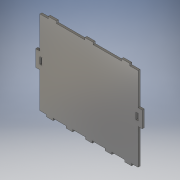
# Autodesk Inventor part: 1-8inch_Middle_2-Parts
Saved by Autodesk Inventor 2018 (Build 220112000, 112)
## iProperties
Created: 2018-01-26
Part Number: 1-8inch_Middle_2-Parts
Material: Generic
Document SubType Name: Modeling
Designer: Olivier
Density: 1 g/cm^3
Appearance: Default
Author: Olivier
Autodesk Inventor part; units mm, degrees
ref_plane "YZ Plane" through (0, 0, 0) normal (1, 0, 0) x (0, 1, 0)
ref_plane "XZ Plane" through (0, 0, 0) normal (0, 1, 0) x (-1, 0, 0)
ref_plane "XY Plane" through (0, 0, 0) normal (0, 0, 1) x (1, 0, 0)
sketch "Sketch1" plane through (0, 0, 0) normal (0, 0, 1) x (1, 0, 0)
  line L0 (-0.5, -5) -> (2.5, -5)
  line L1 (2.5, 5) -> (-0.5, 5)
  line L2 (-0.5, 5) -> (-0.5, -5)
  line L3 (-0.5, 12.5) -> (-0.5, 61.825)
  line L4 (19, 65) -> (24.9, 65)
  line L5 (69, 65) -> (79, 65)
  line L6 (124.9125, 65) -> (129, 65)
  line L7 (150.3125, 12.5) -> (154.5, 12.5)
  line L8 (154.5, -12.5) -> (150.3125, -12.5)
  line L9 (139, -70) -> (129.9925, -70)
  line L10 (109, -70) -> (99.9094, -70)
  line L11 (79, -70) -> (69.8262, -70)
  line L12 (49, -70) -> (39.7431, -70)
  line L13 (19, -70) -> (9.66, -70)
  line L14 (-0.5, -66.825) -> (-0.5, -12.5)
  line L15 (-0.5, -12.5) -> (-6.5, -12.5)
  line L16 (-6.5, 12.5) -> (-0.5, 12.5)
  line L17 (-0.5, -5) -> (2.5, -5)
  line L18 (2.5, 5) -> (-0.5, 5)
  line L19 (-0.5, 5) -> (-0.5, -5)
  line L20 (-0.5, 12.5) -> (-0.5, 61.825)
  line L21 (19, 65) -> (24.9, 65)
  line L22 (69, 65) -> (79, 65)
  line L23 (124.9125, 65) -> (129, 65)
  line L24 (150.3125, 12.5) -> (154.5, 12.5)
  line L25 (154.5, -12.5) -> (150.3125, -12.5)
  line L26 (139, -70) -> (129.9925, -70)
  line L27 (109, -70) -> (99.9094, -70)
  line L28 (79, -70) -> (69.8262, -70)
  line L29 (49, -70) -> (39.7431, -70)
  line L30 (19, -70) -> (9.66, -70)
  line L31 (-0.5, -66.825) -> (-0.5, -12.5)
  line L32 (-0.5, -12.5) -> (-6.5, -12.5)
  line L33 (-6.5, 12.5) -> (-0.5, 12.5)
  line L34 (150.3125, 12.5) -> (156.6625, 12.5)
  line L35 (156.6625, 12.5) -> (156.6625, -12.5)
  line L36 (156.6625, -12.5) -> (150.3125, -12.5)
  line L37 (-0.5, 12.5) -> (-6.85, 12.5)
  line L38 (-6.85, 12.5) -> (-6.85, -12.5)
  line L39 (-6.85, -12.5) -> (-0.5, -12.5)
  line L40 (-0.5, -5) -> (-0.5, 5)
  line L41 (-0.5, 5) -> (2.675, 5)
  line L42 (2.675, 5) -> (2.675, -5)
  line L43 (2.675, -5) -> (-0.5, -5)
  line L44 (-0.5, -5) -> (-0.5, 5)
  line L45 (-0.5, 12.5) -> (-0.5, 61.825)
  line L46 (-0.5, -66.825) -> (-0.5, -12.5)
  line L47 (-0.5, -5) -> (-0.5, 5)
  line L48 (150.3125, 61.825) -> (150.3125, 12.5)
  line L49 (150.3125, -12.5) -> (150.3125, -66.825)
  line L50 (148.5, 5) -> (150.3125, 5)
  line L51 (150.3125, 5) -> (150.3125, -5)
  line L52 (150.3125, -5) -> (148.5, -5)
  line L53 (150.3125, 5) -> (147.1375, 5)
  line L54 (147.1375, 5) -> (147.1375, -5)
  line L55 (147.1375, -5) -> (150.3125, -5)
  line L56 (150.3125, -5) -> (150.3125, 5)
  line L57 (150.3125, 61.825) -> (150.3125, 52.6231)
  line L58 (-0.5, 52.6231) -> (-0.5, 61.825)
  line L59 (150.3125, -66.825) -> (150.3125, -55.7808)
  line L60 (-0.5, -55.7808) -> (-0.5, -66.825)
  line L61 (-0.5, 61.825) -> (12.2, 61.825)
  line L62 (12.2, 61.825) -> (12.2, 65)
  line L63 (12.2, 65) -> (24.9, 65)
  line L64 (24.9, 65) -> (24.9, 61.825)
  line L65 (24.9, 61.825) -> (68.5562, 61.825)
  line L66 (68.5562, 61.825) -> (68.5562, 65)
  line L67 (68.5562, 65) -> (81.2562, 65)
  line L68 (81.2562, 65) -> (81.2562, 61.825)
  line L69 (81.2562, 61.825) -> (124.9125, 61.825)
  line L70 (124.9125, 61.825) -> (124.9125, 65)
  line L71 (124.9125, 65) -> (137.6125, 65)
  line L72 (137.6125, 65) -> (137.6125, 61.825)
  line L73 (137.6125, 61.825) -> (150.3125, 61.825)
  line L74 (124.9125, 65) -> (137.6125, 65)
  line L75 (12.2, 65) -> (24.9, 65)
  line L76 (68.5562, 65) -> (81.2562, 65)
  line L77 (9.66, -70) -> (9.66, -66.825)
  line L78 (9.66, -66.825) -> (-0.5, -66.825)
  line L79 (9.66, -70) -> (19.82, -70)
  line L80 (19.82, -70) -> (19.82, -66.825)
  line L81 (9.66, -66.825) -> (9.66, -70)
  line L82 (19.82, -66.825) -> (39.7431, -66.825)
  line L83 (39.7431, -66.825) -> (39.7431, -70)
  line L84 (19.82, -70) -> (19.82, -66.825)
  line L85 (39.7431, -70) -> (49.9031, -70)
  line L86 (49.9031, -70) -> (49.9031, -66.825)
  line L87 (39.7431, -66.825) -> (39.7431, -70)
  line L88 (69.8262, -70) -> (69.8262, -66.825)
  line L89 (69.8262, -66.825) -> (49.9031, -66.825)
  line L90 (49.9031, -66.825) -> (49.9031, -70)
  line L91 (79.9862, -66.825) -> (79.9862, -70)
  line L92 (79.9862, -70) -> (69.8262, -70)
  line L93 (69.8262, -70) -> (69.8262, -66.825)
  line L94 (79.9862, -66.825) -> (99.9094, -66.825)
  line L95 (99.9094, -66.825) -> (99.9094, -70)
  line L96 (79.9862, -70) -> (79.9862, -66.825)
  line L97 (110.0694, -66.825) -> (110.0694, -70)
  line L98 (110.0694, -70) -> (99.9094, -70)
  line L99 (99.9094, -70) -> (99.9094, -66.825)
  line L100 (110.0694, -66.825) -> (129.9925, -66.825)
  line L101 (129.9925, -66.825) -> (129.9925, -70)
  line L102 (110.0694, -70) -> (110.0694, -66.825)
  line L103 (140.1525, -66.825) -> (140.1525, -70)
  line L104 (140.1525, -70) -> (129.9925, -70)
  line L105 (129.9925, -70) -> (129.9925, -66.825)
  line L106 (140.1525, -66.825) -> (150.3125, -66.825)
  line L107 (140.1525, -70) -> (140.1525, -66.825)
  line L108 (9.66, -66.825) -> (-0.5, -66.825)
  line L109 (-0.5, 61.825) -> (12.2, 61.825)
  line L110 (24.9, 61.825) -> (68.5562, 61.825)
  line L111 (81.2562, 61.825) -> (124.9125, 61.825)
  line L112 (137.6125, 61.825) -> (150.3125, 61.825)
  line L113 (9.66, -70) -> (19.82, -70)
  line L114 (9.66, -70) -> (19.82, -70)
  line L115 (39.7431, -70) -> (49.9031, -70)
  line L116 (39.7431, -70) -> (49.9031, -70)
  line L117 (69.8262, -66.825) -> (49.9031, -66.825)
  line L118 (69.8262, -70) -> (79.9862, -70)
  line L119 (69.8262, -70) -> (79.9862, -70)
  line L120 (99.9094, -66.825) -> (79.9862, -66.825)
  line L121 (99.9094, -70) -> (110.0694, -70)
  line L122 (129.9925, -70) -> (140.1525, -70)
  line L123 (99.9094, -70) -> (110.0694, -70)
  line L124 (129.9925, -70) -> (140.1525, -70)
  line L125 (150.3125, -66.825) -> (140.1525, -66.825)
  line L126 (129.9925, -66.825) -> (110.0694, -66.825)
  line L127 (140.1525, -66.825) -> (150.3125, -66.825)
  dimension "d1" = 6.35
  dimension "d2" = 6.35
  dimension "d3" = 3.175
  dimension "d4" = 3.175
  dimension "d6" = 12.7
  dimension "d7" = 12.7
  dimension "d8" = 43.6562
  dimension "d9" = 12.7
  dimension "d10" = 43.6562
  dimension "d11" = 12.7
  dimension "d12" = 12.7
  dimension "d14" = 10.16
  dimension "d15" = 10.16
  dimension "d16" = 19.9231
  dimension "d18" = 19.9231
  dimension "d19" = 10.16
  dimension "d20" = 19.9231
  dimension "d21" = 10.16
  dimension "d22" = 19.9231
  dimension "d23" = 10.16
  dimension "d25" = 10.16
  constraints: 256 end point, 50 parallel, 43 perpendicular, 25 horizontal, 3 point on line, 1 collinear
  measures "d1" distance of L8.end L35.end
  measures "d2" distance of L14.end L38.end
  measures "d3" distance of L0.start L42.end
  measures "d4" distance of L55.end L54.end
  measures "d6" distance of L3.end L61.end
  measures "d7" distance of L62.end L4.end
  measures "d8" distance of L64.end L65.end
  measures "d9" distance of L66.end L67.end
  measures "d10" distance of L68.end L69.end
  measures "d11" distance of L71.end L6.start
  measures "d12" distance of L48.start L72.end
  measures "d14" distance of L77.end L14.start
  measures "d15" distance of L77.end L80.end
  measures "d16" distance of L12.end L79.end
  measures "d18" distance of L86.end L88.end
  measures "d19" distance of L91.end L11.end
  measures "d20" distance of L10.end L91.end
  measures "d21" distance of L97.end L10.end
  measures "d22" distance of L9.end L97.end
  measures "d23" distance of L103.end L9.end
  measures "d25" distance of L103.start L49.end
extrude "Extrusion1" add sketch "Sketch1" along normal blind 3.175
body "Solid1"
